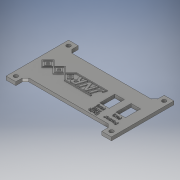
# Autodesk Inventor part: MapleMiniCase_TopCover
Saved by Autodesk Inventor 2018 (Build 220112000, 112)
## iProperties
Created: 2019-01-14
Part Number: MapleMiniCase_TopCover
Material: Generic
Document SubType Name: Modeling
Designer: tbrow
Density: 1 g/cm^3
Appearance: Default
Author: tbrow
## iProperties of the stored document MapleMiniCase_TopCover_3DPrint.ipt
Created: 2019-01-15
Part Number: MapleMiniCase_TopCover_3DPrint
Material: Generic
Document SubType Name: Modeling
Designer: tbrow
Density: 1 g/cm^3
Appearance: Default
Author: tbrow
Autodesk Inventor part; units mm, degrees
ref_plane "YZ Plane" through (0, 0, 0) normal (1, 0, 0) x (0, 1, 0)
ref_plane "XZ Plane" through (0, 0, 0) normal (0, 1, 0) x (-1, 0, 0)
ref_plane "XY Plane" through (0, 0, 0) normal (0, 0, 1) x (1, 0, 0)
sketch "Sketch1" plane through (0, 0, 0) normal (0, 1, 0) x (-1, 0, 0)
  line L0 (0, 0) -> (9.144, 0)
  line L1 (9.144, 0) -> (9.144, -9.144)
  line L2 (9.144, -9.144) -> (89.916, -9.144)
  line L3 (89.916, -9.144) -> (89.916, 0)
  line L4 (89.916, 0) -> (99.06, 0)
  line L5 (99.06, 0) -> (99.06, -58.6994)
  line L6 (99.06, -58.6994) -> (89.916, -58.6994)
  line L7 (89.916, -58.6994) -> (89.916, -49.5554)
  line L8 (89.916, -49.5554) -> (9.144, -49.5554)
  line L9 (9.144, -49.5554) -> (9.144, -58.6994)
  line L10 (9.144, -58.6994) -> (0, -58.6994)
  line L11 (0, -58.6994) -> (0, 0)
  dimension "d0" = 58.6994
  dimension "d1" = 9.144
  dimension "d2" = 9.144
  dimension "d3" = 9.144
  dimension "d4" = 9.144
  dimension "d5" = 9.144
  dimension "d7" = 9.144
  dimension "d16" = 99.06
  constraints: 24 end point, 8 perpendicular, 4 point on line, 2 horizontal
  measures "d0" distance of L4.end L5.end
  measures "d1" distance of L3.end L4.end
  measures "d2" distance of L2.end L3.end
  measures "d3" distance of L6.end L7.end
  measures "d4" distance of L0.start L0.end
  measures "d5" distance of L9.end L10.end
  measures "d7" distance of L5.end L6.end
  measures "d16" distance between parallel lines of L11 L5
extrude "Extrusion1" add sketch "Sketch1" along normal blind 3.175
sketch "Sketch2" plane through (0, 3.175, 0) normal (0, 1, 0) x (1, 0, 0)
  line L0 (-99.06, 0) -> (-89.916, 0) projected
  line L1 (-89.916, 58.6994) -> (-99.06, 58.6994) projected
  line L2 (-89.916, 49.5554) -> (-89.916, 58.6994) projected
  line L3 (-89.916, 0) -> (-89.916, 9.144) projected
  line L4 (-9.144, 0) -> (0, 0) projected
  line L5 (-9.144, 9.144) -> (-9.144, 0) projected
  line L6 (-9.144, 58.6994) -> (-9.144, 49.5554) projected
  circle A0 centre (-94.488, 4.572) radius 1.8542
  circle A1 centre (-94.488, 54.102) radius 1.8542
  circle A2 centre (-4.572, 54.102) radius 1.8542
  circle A3 centre (-4.572, 4.572) radius 1.8542
  line L7 (-99.06, 58.6994) -> (-99.06, 0) projected
  line L8 (0, 58.6994) -> (-9.144, 58.6994) projected
  line L9 (0, 0) -> (0, 58.6994) projected
  dimension "d10" = 3.7084
  dimension "d11" = 3.7084
  dimension "d12" = 3.7084
  dimension "d13" = 3.7084
  dimension "d17" = 4.572
  dimension "d18" = 4.5974
  dimension "d19" = 4.572
  dimension "d20" = 4.572
  dimension "d21" = 4.5974
  dimension "d22" = 4.572
  dimension "d23" = 4.572
  dimension "d24" = 4.572
  constraints: 4 centre point
  measures "d10" diameter of A0
  measures "d11" diameter of A1
  measures "d12" diameter of A2
  measures "d13" diameter of A3
  measures "d17" distance from line of L2 A1.centre
  measures "d18" distance from line of L1 A1.centre
  measures "d19" distance from line of L7 A0.centre
  measures "d20" distance from line of L0 A0.centre
  measures "d21" distance from line of L8 A2.centre
  measures "d22" distance from line of L9 A2.centre
  measures "d23" distance from line of L9 A3.centre
  measures "d24" distance from line of L4 A3.centre
extrude "Extrusion2" cut sketch "Sketch2" against normal blind 25.4
sketch "Sketch3" plane through (0, 3.175, 0) normal (0, 1, 0) x (1, 0, 0)
  line L0 (-33.274, 36.4617) -> (-24.384, 36.4617)
  line L1 (-24.384, 36.4617) -> (-24.384, 22.2377)
  line L2 (-24.384, 22.2377) -> (-33.274, 22.2377)
  line L3 (-33.274, 22.2377) -> (-33.274, 36.4617)
  line L4 (-18.034, 36.4617) -> (-9.144, 36.4617)
  line L5 (-9.144, 36.4617) -> (-9.144, 22.2377)
  line L6 (-9.144, 22.2377) -> (-18.034, 22.2377)
  line L7 (-18.034, 22.2377) -> (-18.034, 36.4617)
  line L8 (0, 0) -> (0, 58.6994) projected
  line L9 (0, 29.3497) -> (-99.06, 29.3497) construction
  line L10 (-99.06, 58.6994) -> (-99.06, 0) projected
  line L11 (-33.274, 29.3497) -> (-24.384, 29.3497) construction
  line L12 (-9.144, 29.3497) -> (-18.034, 29.3497) construction
  dimension "d25" = 14.224
  dimension "d26" = 8.89
  dimension "d27" = 8.89
  dimension "d28" = 6.35
  dimension "d32" = 9.144
  constraints: 22 end point, 6 midpoint, 4 parallel, 2 horizontal, 2 perpendicular, 2 point on line, 1 collinear
  measures "d25" distance of L2.end L0.start
  measures "d26" distance of L0.start L0.end
  measures "d27" distance of L4.start L4.end
  measures "d28" distance between parallel lines of L7 L1
  measures "d32" distance between parallel lines of L8 L5
extrude "Extrusion3" cut sketch "Sketch3" against normal blind 25.4
sketch "Sketch5" plane through (0, 3.175, 0) normal (0, 1, 0) x (1, 0, 0)
  line L0 (-6.9163, 11.6778) -> (-20.2617, 11.6778) construction
  line L1 (-20.2617, 11.6778) -> (-20.2617, 14.6888) construction
  line L2 (-20.2617, 14.6888) -> (-6.9163, 14.6888) construction
  line L3 (-6.9163, 14.6888) -> (-6.9163, 11.6778) construction
  line L4 (-24.384, 22.2377) -> (-33.274, 22.2377) projected
  line L5 (-13.589, 11.6778) -> (-13.589, 11.613) construction
  line L6 (-18.034, 22.2377) -> (-9.144, 22.2377) projected
  line L7 (-13.589, 22.2377) -> (-13.589, 19.0879) construction
  line L8 (-10.6511, 22.2377) -> (-10.6511, 9.144) construction
  line L9 (-89.916, 9.144) -> (-9.144, 9.144) projected
  line L10 (-10.6511, 15.6909) -> (6.071, 15.6909) construction
  line L11 (-24.3341, 10.4275) -> (-33.3239, 10.4275) construction
  line L12 (-33.3239, 10.4275) -> (-33.3239, 17.0935) construction
  line L13 (-33.3239, 17.0935) -> (-24.3341, 17.0935) construction
  line L14 (-24.3341, 17.0935) -> (-24.3341, 10.4275) construction
  line L15 (-33.274, 22.2377) -> (-33.274, 36.4617) projected
  line L16 (-28.829, 10.4275) -> (-28.829, 6.1852) construction
  line L17 (-33.274, 22.2377) -> (-24.384, 22.2377) projected
  line L18 (-28.829, 22.2377) -> (-28.829, 19.0879) construction
  line L19 (-10.5884, 17.4665) -> (-16.5896, 17.4665) construction
  line L20 (-16.5896, 17.4665) -> (-16.5896, 19.3689) construction
  line L21 (-16.5896, 19.3689) -> (-10.5884, 19.3689) construction
  line L22 (-10.5884, 19.3689) -> (-10.5884, 17.4665) construction
  line L23 (-13.589, 17.4665) -> (-13.589, 15.0559) construction
  line L24 (-26.266, 17.4665) -> (-31.392, 17.4665) construction
  line L25 (-31.392, 17.4665) -> (-31.392, 20.1702) construction
  line L26 (-31.392, 20.1702) -> (-26.266, 20.1702) construction
  line L27 (-26.266, 20.1702) -> (-26.266, 17.4665) construction
  line L28 (-28.829, 17.4665) -> (-28.829, 17.4255) construction
  spline S0 degree 2 poles (-9.8961, 12.5585) (-9.8961, 12.7532) (-9.7716, 13.1065) (-9.6561, 13.2242) knots 0 0 0 1 2 2 2
  spline S1 degree 2 poles (-9.6561, 13.2242) (-9.5859, 13.2989) (-9.4138, 13.4212) (-9.312, 13.4642) knots 0 0 0 1 2 2 2
  spline S2 degree 2 poles (-9.312, 13.4642) (-9.2078, 13.5072) (-8.9655, 13.557) (-8.8161, 13.557) knots 0 0 0 1 2 2 2
  line L29 (-8.8161, 13.557) -> (-8.4493, 13.557)
  line L30 (-8.4493, 13.557) -> (-8.4493, 14.4718)
  line L31 (-8.4493, 14.4718) -> (-7.7474, 14.4718)
  line L32 (-7.7474, 14.4718) -> (-7.7474, 11.6778)
  line L33 (-7.7474, 11.6778) -> (-8.832, 11.6778)
  spline S3 degree 2 poles (-8.832, 11.6778) (-9.072, 11.6778) (-9.4229, 11.7661) (-9.5655, 11.8612) knots 0 0 0 1 2 2 2
  spline S4 degree 2 poles (-9.5655, 11.8612) (-9.724, 11.9676) (-9.8961, 12.3163) (-9.8961, 12.5585) knots 0 0 0 1 2 2 2
  spline S5 degree 2 poles (-9.1761, 12.5766) (-9.1761, 12.4566) (-9.0629, 12.2868) (-8.9859, 12.2551) knots 0 0 0 1 2 2 2
  spline S6 degree 2 poles (-8.9859, 12.2551) (-8.8863, 12.2121) (-8.7052, 12.1985) (-8.5489, 12.1985) knots 0 0 0 1 2 2 2
  line L34 (-8.5489, 12.1985) -> (-8.4493, 12.1985)
  line L35 (-8.4493, 12.1985) -> (-8.4493, 13.0363)
  line L36 (-8.4493, 13.0363) -> (-8.4991, 13.0363)
  spline S7 degree 2 poles (-8.4991, 13.0363) (-8.5965, 13.0363) (-8.7731, 13.0317) (-8.8387, 13.0204) knots 0 0 0 1 2 2 2
  spline S8 degree 2 poles (-8.8387, 13.0204) (-8.8954, 13.0114) (-9.0199, 12.957) (-9.0538, 12.9231) knots 0 0 0 1 2 2 2
  spline S9 degree 2 poles (-9.0538, 12.9231) (-9.1263, 12.8551) (-9.1761, 12.7034) (-9.1761, 12.5766) knots 0 0 0 1 2 2 2
  spline S10 degree 2 poles (-12.2554, 13.4189) (-12.2554, 13.9397) (-11.6871, 14.5374) (-11.1686, 14.5374) knots 0 0 0 1 2 2 2
  spline S11 degree 2 poles (-11.1686, 14.5374) (-10.6524, 14.5374) (-10.0795, 13.9397) (-10.0795, 13.4189) knots 0 0 0 1 2 2 2
  spline S12 degree 2 poles (-10.0795, 13.4189) (-10.0795, 12.8936) (-10.6524, 12.2981) (-11.1686, 12.2981) knots 0 0 0 1 2 2 2
  spline S13 degree 2 poles (-11.1686, 12.2981) (-11.6848, 12.2981) (-12.2554, 12.8959) (-12.2554, 13.4189) knots 0 0 0 1 2 2 2
  spline S14 degree 2 poles (-11.5829, 13.4234) (-11.5829, 13.2355) (-11.5218, 12.9842) (-11.4675, 12.9095) knots 0 0 0 1 2 2 2
  spline S15 degree 2 poles (-11.4675, 12.9095) (-11.4086, 12.8302) (-11.2614, 12.7691) (-11.1686, 12.7691) knots 0 0 0 1 2 2 2
  spline S16 degree 2 poles (-11.1686, 12.7691) (-11.078, 12.7691) (-10.9354, 12.8234) (-10.8765, 12.9004) knots 0 0 0 1 2 2 2
  spline S17 degree 2 poles (-10.8765, 12.9004) (-10.8199, 12.9729) (-10.752, 13.2287) (-10.752, 13.4234) knots 0 0 0 1 2 2 2
  spline S18 degree 2 poles (-10.752, 13.4234) (-10.752, 13.6159) (-10.8154, 13.8536) (-10.8675, 13.9261) knots 0 0 0 1 2 2 2
  spline S19 degree 2 poles (-10.8675, 13.9261) (-10.9195, 13.9985) (-11.078, 14.0665) (-11.1731, 14.0665) knots 0 0 0 1 2 2 2
  spline S20 degree 2 poles (-11.1731, 14.0665) (-11.2524, 14.0665) (-11.4154, 13.9985) (-11.4652, 13.9306) knots 0 0 0 1 2 2 2
  spline S21 degree 2 poles (-11.4652, 13.9306) (-11.5218, 13.8514) (-11.5829, 13.6227) (-11.5829, 13.4234) knots 0 0 0 1 2 2 2
  line L37 (-15.7445, 12.3638) -> (-15.1286, 14.4718)
  line L38 (-15.1286, 14.4718) -> (-14.4313, 14.4718)
  line L39 (-14.4313, 14.4718) -> (-14.0599, 13.1087)
  line L40 (-14.0599, 13.1087) -> (-13.6886, 14.4718)
  line L41 (-13.6886, 14.4718) -> (-12.9913, 14.4718)
  line L42 (-12.9913, 14.4718) -> (-12.3799, 12.3638)
  line L43 (-12.3799, 12.3638) -> (-13.0705, 12.3638)
  line L44 (-13.0705, 12.3638) -> (-13.3943, 13.7585)
  line L45 (-13.3943, 13.7585) -> (-13.7928, 12.3638)
  line L46 (-13.7928, 12.3638) -> (-14.3747, 12.3638)
  line L47 (-14.3747, 12.3638) -> (-14.7505, 13.7585)
  line L48 (-14.7505, 13.7585) -> (-15.0698, 12.3638)
  line L49 (-15.0698, 12.3638) -> (-15.7445, 12.3638)
  spline S22 degree 2 poles (-17.103, 14.5284) (-16.5053, 14.5284) (-15.869, 13.9578) (-15.869, 13.4302) knots 0 0 0 1 2 2 2
  spline S23 degree 2 poles (-15.869, 13.4302) (-15.869, 12.914) (-16.4622, 12.2981) (-16.9966, 12.2981) knots 0 0 0 1 2 2 2
  spline S24 degree 2 poles (-16.9966, 12.2981) (-17.4789, 12.2981) (-17.9679, 12.8212) (-17.9679, 13.3057) knots 0 0 0 1 2 2 2
  line L50 (-17.9679, 13.3057) -> (-17.9679, 13.5434)
  line L51 (-17.9679, 13.5434) -> (-16.5256, 13.5434)
  spline S25 degree 2 poles (-16.5256, 13.5434) (-16.5347, 13.6906) (-16.6411, 13.8853) (-16.7272, 13.9442) knots 0 0 0 1 2 2 2
  spline S26 degree 2 poles (-16.7272, 13.9442) (-16.8109, 14.0031) (-17.0373, 14.0529) (-17.1709, 14.0529) knots 0 0 0 1 2 2 2
  spline S27 degree 2 poles (-17.1709, 14.0529) (-17.2841, 14.0529) (-17.506, 14.0031) (-17.5989, 13.9601) knots 0 0 0 1 2 2 2
  spline S28 degree 2 poles (-17.5989, 13.9601) (-17.6804, 13.9261) (-17.8162, 13.8423) (-17.8592, 13.8106) knots 0 0 0 1 2 2 2
  line L52 (-17.8592, 13.8106) -> (-17.9294, 13.8106)
  line L53 (-17.9294, 13.8106) -> (-17.9294, 14.354)
  spline S29 degree 2 poles (-17.9294, 14.354) (-17.8479, 14.3857) (-17.7166, 14.4401) (-17.5989, 14.4672) knots 0 0 0 1 2 2 2
  spline S30 degree 2 poles (-17.5989, 14.4672) (-17.4924, 14.4967) (-17.266, 14.5284) (-17.103, 14.5284) knots 0 0 0 1 2 2 2
  spline S31 degree 2 poles (-17.3204, 13.1472) (-17.3158, 12.9389) (-17.1324, 12.7193) (-16.9445, 12.7193) knots 0 0 0 1 2 2 2
  spline S32 degree 2 poles (-16.9445, 12.7193) (-16.7521, 12.7193) (-16.5347, 12.9502) (-16.5234, 13.1472) knots 0 0 0 1 2 2 2
  line L54 (-16.5234, 13.1472) -> (-17.3204, 13.1472)
  line L55 (-19.7204, 12.9865) -> (-19.6661, 12.9865)
  spline S33 degree 2 poles (-19.6661, 12.9865) (-19.6276, 12.9729) (-19.4849, 12.9593) (-19.3989, 12.9593) knots 0 0 0 1 2 2 2
  spline S34 degree 2 poles (-19.3989, 12.9593) (-19.297, 12.9593) (-19.0683, 13.0204) (-18.9619, 13.0612) knots 0 0 0 1 2 2 2
  line L56 (-18.9619, 13.0612) -> (-18.9619, 14.4718)
  line L57 (-18.9619, 14.4718) -> (-18.3053, 14.4718)
  line L58 (-18.3053, 14.4718) -> (-18.3053, 12.3638)
  line L59 (-18.3053, 12.3638) -> (-18.9619, 12.3638)
  line L60 (-18.9619, 12.3638) -> (-18.9619, 12.6672)
  spline S35 degree 2 poles (-18.9619, 12.6672) (-19.0072, 12.6265) (-19.1657, 12.4997) (-19.2313, 12.4612) knots 0 0 0 1 2 2 2
  spline S36 degree 2 poles (-19.2313, 12.4612) (-19.3038, 12.4181) (-19.494, 12.357) (-19.5778, 12.357) knots 0 0 0 1 2 2 2
  spline S37 degree 2 poles (-19.5778, 12.357) (-19.6095, 12.357) (-19.6887, 12.3615) (-19.7204, 12.3638) knots 0 0 0 1 2 2 2
  line L61 (-19.7204, 12.3638) -> (-19.7204, 12.9865)
  line L62 (-11.1842, 20.3183) -> (-10.6523, 20.3183)
  spline S38 degree 2 poles (-10.6523, 20.3183) (-10.5298, 20.1713) (-10.3286, 19.8616) (-10.2569, 19.6832) knots 0 0 0 1 2 2 2
  spline S39 degree 2 poles (-10.2569, 19.6832) (-10.1887, 19.517) (-10.1117, 19.1111) (-10.1117, 18.8924) knots 0 0 0 1 2 2 2
  spline S40 degree 2 poles (-10.1117, 18.8924) (-10.1117, 18.6527) (-10.1922, 18.2643) (-10.2551, 18.1033) knots 0 0 0 1 2 2 2
  spline S41 degree 2 poles (-10.2551, 18.1033) (-10.3251, 17.9283) (-10.5263, 17.6169) (-10.6523, 17.4665) knots 0 0 0 1 2 2 2
  line L63 (-10.6523, 17.4665) -> (-11.1842, 17.4665)
  line L64 (-11.1842, 17.4665) -> (-11.1842, 17.5084)
  spline S42 degree 2 poles (-11.1842, 17.5084) (-11.067, 17.6134) (-10.8535, 17.8829) (-10.7625, 18.0613) knots 0 0 0 1 2 2 2
  spline S43 degree 2 poles (-10.7625, 18.0613) (-10.675, 18.2345) (-10.5666, 18.6544) (-10.5666, 18.8924) knots 0 0 0 1 2 2 2
  spline S44 degree 2 poles (-10.5666, 18.8924) (-10.5666, 19.1408) (-10.6716, 19.5432) (-10.7625, 19.7234) knots 0 0 0 1 2 2 2
  spline S45 degree 2 poles (-10.7625, 19.7234) (-10.85, 19.8931) (-11.0687, 20.1731) (-11.1842, 20.2763) knots 0 0 0 1 2 2 2
  line L65 (-11.1842, 20.2763) -> (-11.1842, 20.3183)
  spline S46 degree 2 poles (-13.4901, 18.6422) (-13.4901, 19.1671) (-12.9303, 19.7672) (-12.4439, 19.7672) knots 0 0 0 1 2 2 2
  spline S47 degree 2 poles (-12.4439, 19.7672) (-11.9558, 19.7672) (-11.3994, 19.1601) (-11.3994, 18.6422) knots 0 0 0 1 2 2 2
  spline S48 degree 2 poles (-11.3994, 18.6422) (-11.3994, 18.1226) (-11.9558, 17.5172) (-12.4439, 17.5172) knots 0 0 0 1 2 2 2
  spline S49 degree 2 poles (-12.4439, 17.5172) (-12.9303, 17.5172) (-13.4901, 18.1191) (-13.4901, 18.6422) knots 0 0 0 1 2 2 2
  spline S50 degree 2 poles (-12.9303, 18.6422) (-12.9303, 18.448) (-12.8515, 18.1768) (-12.7833, 18.0911) knots 0 0 0 1 2 2 2
  spline S51 degree 2 poles (-12.7833, 18.0911) (-12.7151, 18.0018) (-12.5401, 17.9248) (-12.4456, 17.9248) knots 0 0 0 1 2 2 2
  spline S52 degree 2 poles (-12.4456, 17.9248) (-12.3459, 17.9248) (-12.1832, 17.9966) (-12.108, 18.0876) knots 0 0 0 1 2 2 2
  spline S53 degree 2 poles (-12.108, 18.0876) (-12.0415, 18.1715) (-11.9593, 18.4497) (-11.9593, 18.6422) knots 0 0 0 1 2 2 2
  spline S54 degree 2 poles (-11.9593, 18.6422) (-11.9593, 18.8416) (-12.038, 19.1041) (-12.1062, 19.1933) knots 0 0 0 1 2 2 2
  spline S55 degree 2 poles (-12.1062, 19.1933) (-12.1745, 19.2825) (-12.3512, 19.3595) (-12.4456, 19.3595) knots 0 0 0 1 2 2 2
  spline S56 degree 2 poles (-12.4456, 19.3595) (-12.5419, 19.3595) (-12.7203, 19.2773) (-12.7851, 19.1898) knots 0 0 0 1 2 2 2
  spline S57 degree 2 poles (-12.7851, 19.1898) (-12.855, 19.0953) (-12.9303, 18.8451) (-12.9303, 18.6422) knots 0 0 0 1 2 2 2
  line L66 (-15.6614, 19.7217) -> (-15.14, 19.7217)
  line L67 (-15.14, 19.7217) -> (-14.3072, 18.217)
  line L68 (-14.3072, 18.217) -> (-14.3072, 19.7217)
  line L69 (-14.3072, 19.7217) -> (-13.8121, 19.7217)
  line L70 (-13.8121, 19.7217) -> (-13.8121, 17.5627)
  line L71 (-13.8121, 17.5627) -> (-14.4769, 17.5627)
  line L72 (-14.4769, 17.5627) -> (-15.1663, 18.7996)
  line L73 (-15.1663, 18.7996) -> (-15.1663, 17.5627)
  line L74 (-15.1663, 17.5627) -> (-15.6614, 17.5627)
  line L75 (-15.6614, 17.5627) -> (-15.6614, 19.7217)
  spline S58 degree 2 poles (-17.0628, 18.8924) (-17.0628, 19.1111) (-16.9858, 19.5152) (-16.9176, 19.6832) knots 0 0 0 1 2 2 2
  spline S59 degree 2 poles (-16.9176, 19.6832) (-16.8459, 19.8616) (-16.6447, 20.1713) (-16.5222, 20.3183) knots 0 0 0 1 2 2 2
  line L76 (-16.5222, 20.3183) -> (-15.9903, 20.3183)
  line L77 (-15.9903, 20.3183) -> (-15.9903, 20.2763)
  spline S60 degree 2 poles (-15.9903, 20.2763) (-16.1058, 20.1731) (-16.3262, 19.8949) (-16.412, 19.7234) knots 0 0 0 1 2 2 2
  spline S61 degree 2 poles (-16.412, 19.7234) (-16.503, 19.5432) (-16.6079, 19.1408) (-16.6079, 18.8924) knots 0 0 0 1 2 2 2
  spline S62 degree 2 poles (-16.6079, 18.8924) (-16.6079, 18.6544) (-16.4995, 18.2345) (-16.412, 18.0613) knots 0 0 0 1 2 2 2
  spline S63 degree 2 poles (-16.412, 18.0613) (-16.321, 17.8829) (-16.1075, 17.6134) (-15.9903, 17.5084) knots 0 0 0 1 2 2 2
  line L78 (-15.9903, 17.5084) -> (-15.9903, 17.4665)
  line L79 (-15.9903, 17.4665) -> (-16.5222, 17.4665)
  spline S64 degree 2 poles (-16.5222, 17.4665) (-16.6482, 17.6169) (-16.8494, 17.9283) (-16.9194, 18.1033) knots 0 0 0 1 2 2 2
  spline S65 degree 2 poles (-16.9194, 18.1033) (-16.9823, 18.2643) (-17.0628, 18.6527) (-17.0628, 18.8924) knots 0 0 0 1 2 2 2
  line L80 (-26.4242, 20.3183) -> (-25.8923, 20.3183)
  spline S66 degree 2 poles (-25.8923, 20.3183) (-25.7698, 20.1713) (-25.5686, 19.8616) (-25.4969, 19.6832) knots 0 0 0 1 2 2 2
  spline S67 degree 2 poles (-25.4969, 19.6832) (-25.4287, 19.517) (-25.3517, 19.1111) (-25.3517, 18.8924) knots 0 0 0 1 2 2 2
  spline S68 degree 2 poles (-25.3517, 18.8924) (-25.3517, 18.6527) (-25.4322, 18.2643) (-25.4951, 18.1033) knots 0 0 0 1 2 2 2
  spline S69 degree 2 poles (-25.4951, 18.1033) (-25.5651, 17.9283) (-25.7663, 17.6169) (-25.8923, 17.4665) knots 0 0 0 1 2 2 2
  line L81 (-25.8923, 17.4665) -> (-26.4242, 17.4665)
  line L82 (-26.4242, 17.4665) -> (-26.4242, 17.5084)
  spline S70 degree 2 poles (-26.4242, 17.5084) (-26.307, 17.6134) (-26.0935, 17.8829) (-26.0025, 18.0613) knots 0 0 0 1 2 2 2
  spline S71 degree 2 poles (-26.0025, 18.0613) (-25.915, 18.2345) (-25.8066, 18.6544) (-25.8066, 18.8924) knots 0 0 0 1 2 2 2
  spline S72 degree 2 poles (-25.8066, 18.8924) (-25.8066, 19.1408) (-25.9116, 19.5432) (-26.0025, 19.7234) knots 0 0 0 1 2 2 2
  spline S73 degree 2 poles (-26.0025, 19.7234) (-26.09, 19.8931) (-26.3087, 20.1731) (-26.4242, 20.2763) knots 0 0 0 1 2 2 2
  line L83 (-26.4242, 20.2763) -> (-26.4242, 20.3183)
  spline S74 degree 2 poles (-28.7301, 18.6422) (-28.7301, 19.1671) (-28.1703, 19.7672) (-27.6839, 19.7672) knots 0 0 0 1 2 2 2
  spline S75 degree 2 poles (-27.6839, 19.7672) (-27.1958, 19.7672) (-26.6394, 19.1601) (-26.6394, 18.6422) knots 0 0 0 1 2 2 2
  spline S76 degree 2 poles (-26.6394, 18.6422) (-26.6394, 18.1226) (-27.1958, 17.5172) (-27.6839, 17.5172) knots 0 0 0 1 2 2 2
  spline S77 degree 2 poles (-27.6839, 17.5172) (-28.1703, 17.5172) (-28.7301, 18.1191) (-28.7301, 18.6422) knots 0 0 0 1 2 2 2
  spline S78 degree 2 poles (-28.1703, 18.6422) (-28.1703, 18.448) (-28.0915, 18.1768) (-28.0233, 18.0911) knots 0 0 0 1 2 2 2
  spline S79 degree 2 poles (-28.0233, 18.0911) (-27.9551, 18.0018) (-27.7801, 17.9248) (-27.6856, 17.9248) knots 0 0 0 1 2 2 2
  spline S80 degree 2 poles (-27.6856, 17.9248) (-27.5859, 17.9248) (-27.4232, 17.9966) (-27.348, 18.0876) knots 0 0 0 1 2 2 2
  spline S81 degree 2 poles (-27.348, 18.0876) (-27.2815, 18.1715) (-27.1993, 18.4497) (-27.1993, 18.6422) knots 0 0 0 1 2 2 2
  spline S82 degree 2 poles (-27.1993, 18.6422) (-27.1993, 18.8416) (-27.278, 19.1041) (-27.3462, 19.1933) knots 0 0 0 1 2 2 2
  spline S83 degree 2 poles (-27.3462, 19.1933) (-27.4145, 19.2825) (-27.5912, 19.3595) (-27.6856, 19.3595) knots 0 0 0 1 2 2 2
  spline S84 degree 2 poles (-27.6856, 19.3595) (-27.7819, 19.3595) (-27.9603, 19.2773) (-28.0251, 19.1898) knots 0 0 0 1 2 2 2
  spline S85 degree 2 poles (-28.0251, 19.1898) (-28.095, 19.0953) (-28.1703, 18.8451) (-28.1703, 18.6422) knots 0 0 0 1 2 2 2
  line L84 (-30.9014, 19.7217) -> (-30.38, 19.7217)
  line L85 (-30.38, 19.7217) -> (-29.5472, 18.217)
  line L86 (-29.5472, 18.217) -> (-29.5472, 19.7217)
  line L87 (-29.5472, 19.7217) -> (-29.0521, 19.7217)
  line L88 (-29.0521, 19.7217) -> (-29.0521, 17.5627)
  line L89 (-29.0521, 17.5627) -> (-29.7169, 17.5627)
  line L90 (-29.7169, 17.5627) -> (-30.4063, 18.7996)
  line L91 (-30.4063, 18.7996) -> (-30.4063, 17.5627)
  line L92 (-30.4063, 17.5627) -> (-30.9014, 17.5627)
  line L93 (-30.9014, 17.5627) -> (-30.9014, 19.7217)
  spline S86 degree 2 poles (-32.3028, 18.8924) (-32.3028, 19.1111) (-32.2258, 19.5152) (-32.1576, 19.6832) knots 0 0 0 1 2 2 2
  spline S87 degree 2 poles (-32.1576, 19.6832) (-32.0859, 19.8616) (-31.8847, 20.1713) (-31.7622, 20.3183) knots 0 0 0 1 2 2 2
  line L94 (-31.7622, 20.3183) -> (-31.2303, 20.3183)
  line L95 (-31.2303, 20.3183) -> (-31.2303, 20.2763)
  spline S88 degree 2 poles (-31.2303, 20.2763) (-31.3458, 20.1731) (-31.5662, 19.8949) (-31.652, 19.7234) knots 0 0 0 1 2 2 2
  spline S89 degree 2 poles (-31.652, 19.7234) (-31.743, 19.5432) (-31.8479, 19.1408) (-31.8479, 18.8924) knots 0 0 0 1 2 2 2
  spline S90 degree 2 poles (-31.8479, 18.8924) (-31.8479, 18.6544) (-31.7395, 18.2345) (-31.652, 18.0613) knots 0 0 0 1 2 2 2
  spline S91 degree 2 poles (-31.652, 18.0613) (-31.561, 17.8829) (-31.3475, 17.6134) (-31.2303, 17.5084) knots 0 0 0 1 2 2 2
  line L96 (-31.2303, 17.5084) -> (-31.2303, 17.4665)
  line L97 (-31.2303, 17.4665) -> (-31.7622, 17.4665)
  spline S92 degree 2 poles (-31.7622, 17.4665) (-31.8882, 17.6169) (-32.0894, 17.9283) (-32.1594, 18.1033) knots 0 0 0 1 2 2 2
  spline S93 degree 2 poles (-32.1594, 18.1033) (-32.2223, 18.2643) (-32.3028, 18.6527) (-32.3028, 18.8924) knots 0 0 0 1 2 2 2
  spline S94 degree 2 poles (-27.0584, 11.8268) (-27.0584, 12.2185) (-26.7165, 12.8343) (-26.4561, 12.9996) knots 0 0 0 1 2 2 2
  spline S95 degree 2 poles (-26.4561, 12.9996) (-26.2388, 13.14) (-25.7271, 13.2215) (-25.4395, 13.2215) knots 0 0 0 1 2 2 2
  line L98 (-25.4395, 13.2215) -> (-24.5655, 13.2215)
  line L99 (-24.5655, 13.2215) -> (-24.5655, 10.4275)
  line L100 (-24.5655, 10.4275) -> (-25.4305, 10.4275)
  spline S96 degree 2 poles (-25.4305, 10.4275) (-25.7248, 10.4275) (-26.2388, 10.5022) (-26.4652, 10.6471) knots 0 0 0 1 2 2 2
  spline S97 degree 2 poles (-26.4652, 10.6471) (-26.7392, 10.8237) (-27.0584, 11.4215) (-27.0584, 11.8268) knots 0 0 0 1 2 2 2
  spline S98 degree 2 poles (-26.3384, 11.8222) (-26.3384, 11.546) (-26.1482, 11.152) (-25.9535, 11.0411) knots 0 0 0 1 2 2 2
  spline S99 degree 2 poles (-25.9535, 11.0411) (-25.8108, 10.9641) (-25.4984, 10.9483) (-25.281, 10.9483) knots 0 0 0 1 2 2 2
  line L101 (-25.281, 10.9483) -> (-25.2674, 10.9483)
  line L102 (-25.2674, 10.9483) -> (-25.2674, 12.6985)
  line L103 (-25.2674, 12.6985) -> (-25.281, 12.6985)
  spline S100 degree 2 poles (-25.281, 12.6985) (-25.5165, 12.6985) (-25.8403, 12.6826) (-25.9875, 12.5898) knots 0 0 0 1 2 2 2
  spline S101 degree 2 poles (-25.9875, 12.5898) (-26.1595, 12.4811) (-26.3384, 12.0985) (-26.3384, 11.8222) knots 0 0 0 1 2 2 2
  spline S102 degree 2 poles (-28.5981, 12.9973) (-28.5301, 13.0539) (-28.4237, 13.1445) (-28.3331, 13.1898) knots 0 0 0 1 2 2 2
  spline S103 degree 2 poles (-28.3331, 13.1898) (-28.2448, 13.2328) (-28.0773, 13.2781) (-27.9279, 13.2781) knots 0 0 0 1 2 2 2
  spline S104 degree 2 poles (-27.9279, 13.2781) (-27.6471, 13.2781) (-27.278, 12.9022) (-27.278, 12.617) knots 0 0 0 1 2 2 2
  spline S105 degree 2 poles (-27.278, 12.617) (-27.278, 12.3837) (-27.466, 12.0939) (-27.6426, 12.0102) knots 0 0 0 1 2 2 2
  spline S106 degree 2 poles (-27.6426, 12.0102) (-27.8214, 11.9241) (-28.3173, 11.8562) (-28.6026, 11.8381) knots 0 0 0 1 2 2 2
  line L104 (-28.6026, 11.8381) -> (-28.6026, 11.8268)
  spline S107 degree 2 poles (-28.6026, 11.8268) (-28.6026, 11.6524) (-28.3445, 11.5188) (-28.0863, 11.5188) knots 0 0 0 1 2 2 2
  spline S108 degree 2 poles (-28.0863, 11.5188) (-27.9709, 11.5188) (-27.6584, 11.6026) (-27.5112, 11.6683) knots 0 0 0 1 2 2 2
  line L105 (-27.5112, 11.6683) -> (-27.4546, 11.6683)
  line L106 (-27.4546, 11.6683) -> (-27.4546, 11.1588)
  spline S109 degree 2 poles (-27.4546, 11.1588) (-27.552, 11.1317) (-27.9867, 11.0547) (-28.2086, 11.0547) knots 0 0 0 1 2 2 2
  spline S110 degree 2 poles (-28.2086, 11.0547) (-28.752, 11.0547) (-29.2501, 11.4169) (-29.2501, 11.7883) knots 0 0 0 1 2 2 2
  line L107 (-29.2501, 11.7883) -> (-29.2501, 13.2215)
  line L108 (-29.2501, 13.2215) -> (-28.5981, 13.2215)
  line L109 (-28.5981, 13.2215) -> (-28.5981, 12.9973)
  line L110 (-28.5981, 12.6713) -> (-28.5981, 12.2343)
  spline S111 degree 2 poles (-28.5981, 12.2343) (-28.4305, 12.2502) (-28.2245, 12.2751) (-28.1248, 12.3113) knots 0 0 0 1 2 2 2
  spline S112 degree 2 poles (-28.1248, 12.3113) (-28.0365, 12.3407) (-27.9414, 12.463) (-27.9414, 12.5626) knots 0 0 0 1 2 2 2
  spline S113 degree 2 poles (-27.9414, 12.5626) (-27.9414, 12.7098) (-28.1022, 12.8207) (-28.2584, 12.8207) knots 0 0 0 1 2 2 2
  spline S114 degree 2 poles (-28.2584, 12.8207) (-28.3445, 12.8207) (-28.5256, 12.7415) (-28.5981, 12.6713) knots 0 0 0 1 2 2 2
  spline S115 degree 2 poles (-30.543, 13.2623) (-30.1422, 13.2623) (-29.7754, 12.9317) (-29.7754, 12.5558) knots 0 0 0 1 2 2 2
  line L111 (-29.7754, 12.5558) -> (-29.7754, 11.5709)
  line L112 (-29.7754, 11.5709) -> (-29.5241, 11.5709)
  line L113 (-29.5241, 11.5709) -> (-29.5241, 11.1135)
  line L114 (-29.5241, 11.1135) -> (-29.7754, 11.1135)
  line L115 (-29.7754, 11.1135) -> (-29.7754, 10.5113)
  line L116 (-29.7754, 10.5113) -> (-30.432, 10.5113)
  line L117 (-30.432, 10.5113) -> (-30.432, 11.1135)
  line L118 (-30.432, 11.1135) -> (-31.066, 11.1135)
  line L119 (-31.066, 11.1135) -> (-31.066, 11.5709)
  line L120 (-31.066, 11.5709) -> (-30.432, 11.5709)
  line L121 (-30.432, 11.5709) -> (-30.432, 12.3204)
  spline S116 degree 2 poles (-30.432, 12.3204) (-30.432, 12.4313) (-30.4366, 12.5966) (-30.4637, 12.6622) knots 0 0 0 1 2 2 2
  spline S117 degree 2 poles (-30.4637, 12.6622) (-30.4909, 12.7279) (-30.6245, 12.8049) (-30.7513, 12.8049) knots 0 0 0 1 2 2 2
  spline S118 degree 2 poles (-30.7513, 12.8049) (-30.8056, 12.8049) (-30.9754, 12.7596) (-31.0094, 12.7415) knots 0 0 0 1 2 2 2
  line L122 (-31.0094, 12.7415) -> (-31.066, 12.7415)
  line L123 (-31.066, 12.7415) -> (-31.066, 13.2034)
  spline S119 degree 2 poles (-31.066, 13.2034) (-30.9596, 13.2306) (-30.7196, 13.2623) (-30.543, 13.2623) knots 0 0 0 1 2 2 2
  spline S120 degree 2 poles (-32.4947, 12.9973) (-32.4268, 13.0539) (-32.3204, 13.1445) (-32.2298, 13.1898) knots 0 0 0 1 2 2 2
  spline S121 degree 2 poles (-32.2298, 13.1898) (-32.1415, 13.2328) (-31.9739, 13.2781) (-31.8245, 13.2781) knots 0 0 0 1 2 2 2
  spline S122 degree 2 poles (-31.8245, 13.2781) (-31.5438, 13.2781) (-31.1747, 12.9022) (-31.1747, 12.617) knots 0 0 0 1 2 2 2
  spline S123 degree 2 poles (-31.1747, 12.617) (-31.1747, 12.3837) (-31.3626, 12.0939) (-31.5392, 12.0102) knots 0 0 0 1 2 2 2
  spline S124 degree 2 poles (-31.5392, 12.0102) (-31.7181, 11.9241) (-32.214, 11.8562) (-32.4992, 11.8381) knots 0 0 0 1 2 2 2
  line L124 (-32.4992, 11.8381) -> (-32.4992, 11.8268)
  spline S125 degree 2 poles (-32.4992, 11.8268) (-32.4992, 11.6524) (-32.2411, 11.5188) (-31.983, 11.5188) knots 0 0 0 1 2 2 2
  spline S126 degree 2 poles (-31.983, 11.5188) (-31.8675, 11.5188) (-31.5551, 11.6026) (-31.4079, 11.6683) knots 0 0 0 1 2 2 2
  line L125 (-31.4079, 11.6683) -> (-31.3513, 11.6683)
  line L126 (-31.3513, 11.6683) -> (-31.3513, 11.1588)
  spline S127 degree 2 poles (-31.3513, 11.1588) (-31.4487, 11.1317) (-31.8834, 11.0547) (-32.1053, 11.0547) knots 0 0 0 1 2 2 2
  spline S128 degree 2 poles (-32.1053, 11.0547) (-32.6487, 11.0547) (-33.1468, 11.4169) (-33.1468, 11.7883) knots 0 0 0 1 2 2 2
  line L127 (-33.1468, 11.7883) -> (-33.1468, 13.2215)
  line L128 (-33.1468, 13.2215) -> (-32.4947, 13.2215)
  line L129 (-32.4947, 13.2215) -> (-32.4947, 12.9973)
  line L130 (-32.4947, 12.6713) -> (-32.4947, 12.2343)
  spline S129 degree 2 poles (-32.4947, 12.2343) (-32.3272, 12.2502) (-32.1211, 12.2751) (-32.0215, 12.3113) knots 0 0 0 1 2 2 2
  spline S130 degree 2 poles (-32.0215, 12.3113) (-31.9332, 12.3407) (-31.8381, 12.463) (-31.8381, 12.5626) knots 0 0 0 1 2 2 2
  spline S131 degree 2 poles (-31.8381, 12.5626) (-31.8381, 12.7098) (-31.9989, 12.8207) (-32.1551, 12.8207) knots 0 0 0 1 2 2 2
  spline S132 degree 2 poles (-32.1551, 12.8207) (-32.2411, 12.8207) (-32.4223, 12.7415) (-32.4947, 12.6713) knots 0 0 0 1 2 2 2
  line L131 (-25.2799, 16.0155) -> (-26.2241, 13.2215)
  line L132 (-26.2241, 13.2215) -> (-26.9894, 13.2215)
  line L133 (-26.9894, 13.2215) -> (-27.9335, 16.0155)
  line L134 (-27.9335, 16.0155) -> (-27.2112, 16.0155)
  line L135 (-27.2112, 16.0155) -> (-27.0369, 15.4449)
  line L136 (-27.0369, 15.4449) -> (-26.1584, 15.4449)
  line L137 (-26.1584, 15.4449) -> (-25.9818, 16.0155)
  line L138 (-25.9818, 16.0155) -> (-25.2799, 16.0155)
  line L139 (-26.8829, 14.9377) -> (-26.5976, 14.014)
  line L140 (-26.5976, 14.014) -> (-26.3101, 14.9377)
  line L141 (-26.3101, 14.9377) -> (-26.8829, 14.9377)
  spline S133 degree 2 poles (-29.206, 16.0721) (-28.9456, 16.0721) (-28.5131, 15.9408) (-28.3524, 15.8049) knots 0 0 0 1 2 2 2
  spline S134 degree 2 poles (-28.3524, 15.8049) (-28.1962, 15.6668) (-28.0196, 15.2525) (-28.0196, 14.9717) knots 0 0 0 1 2 2 2
  spline S135 degree 2 poles (-28.0196, 14.9717) (-28.0196, 14.6683) (-28.2097, 14.2449) (-28.375, 14.1091) knots 0 0 0 1 2 2 2
  spline S136 degree 2 poles (-28.375, 14.1091) (-28.5313, 13.9777) (-28.9569, 13.8509) (-29.1879, 13.8509) knots 0 0 0 1 2 2 2
  spline S137 degree 2 poles (-29.1879, 13.8509) (-29.3622, 13.8509) (-29.7109, 13.9324) (-29.8875, 14.0208) knots 0 0 0 1 2 2 2
  line L142 (-29.8875, 14.0208) -> (-29.8875, 14.5823)
  line L143 (-29.8875, 14.5823) -> (-29.8037, 14.5823)
  spline S138 degree 2 poles (-29.8037, 14.5823) (-29.763, 14.5438) (-29.6498, 14.4532) (-29.5818, 14.417) knots 0 0 0 1 2 2 2
  spline S139 degree 2 poles (-29.5818, 14.417) (-29.5094, 14.3762) (-29.3305, 14.3219) (-29.2196, 14.3219) knots 0 0 0 1 2 2 2
  spline S140 degree 2 poles (-29.2196, 14.3219) (-28.9682, 14.3219) (-28.692, 14.6728) (-28.692, 14.9717) knots 0 0 0 1 2 2 2
  spline S141 degree 2 poles (-28.692, 14.9717) (-28.692, 15.2887) (-28.9864, 15.6012) (-29.2309, 15.6012) knots 0 0 0 1 2 2 2
  spline S142 degree 2 poles (-29.2309, 15.6012) (-29.3554, 15.6012) (-29.5411, 15.5445) (-29.609, 15.5038) knots 0 0 0 1 2 2 2
  spline S143 degree 2 poles (-29.609, 15.5038) (-29.6747, 15.4653) (-29.7698, 15.3793) (-29.8037, 15.3453) knots 0 0 0 1 2 2 2
  line L144 (-29.8037, 15.3453) -> (-29.8875, 15.3453)
  line L145 (-29.8875, 15.3453) -> (-29.8875, 15.9091)
  spline S144 degree 2 poles (-29.8875, 15.9091) (-29.8309, 15.934) (-29.6837, 15.9974) (-29.6067, 16.0178) knots 0 0 0 1 2 2 2
  spline S145 degree 2 poles (-29.6067, 16.0178) (-29.5117, 16.0449) (-29.3441, 16.0721) (-29.206, 16.0721) knots 0 0 0 1 2 2 2
  line L146 (-32.1155, 16.7876) -> (-31.4588, 16.7876)
  line L147 (-31.4588, 16.7876) -> (-31.4588, 15.8072)
  spline S146 degree 2 poles (-31.4588, 15.8072) (-31.3887, 15.8638) (-31.2392, 15.9702) (-31.1713, 16.0019) knots 0 0 0 1 2 2 2
  spline S147 degree 2 poles (-31.1713, 16.0019) (-31.0875, 16.0404) (-30.9494, 16.0721) (-30.8317, 16.0721) knots 0 0 0 1 2 2 2
  spline S148 degree 2 poles (-30.8317, 16.0721) (-30.4717, 16.0721) (-30.0505, 15.4766) (-30.0505, 14.9785) knots 0 0 0 1 2 2 2
  spline S149 degree 2 poles (-30.0505, 14.9785) (-30.0505, 14.7023) (-30.1932, 14.297) (-30.3177, 14.1475) knots 0 0 0 1 2 2 2
  spline S150 degree 2 poles (-30.3177, 14.1475) (-30.4332, 14.0094) (-30.7592, 13.8509) (-30.9403, 13.8509) knots 0 0 0 1 2 2 2
  spline S151 degree 2 poles (-30.9403, 13.8509) (-31.0966, 13.8509) (-31.3275, 13.9302) (-31.4543, 14.0026) knots 0 0 0 1 2 2 2
  line L148 (-31.4543, 14.0026) -> (-31.4792, 13.9075)
  line L149 (-31.4792, 13.9075) -> (-32.1155, 13.9075)
  line L150 (-32.1155, 13.9075) -> (-32.1155, 16.7876)
  line L151 (-31.4588, 15.4336) -> (-31.4588, 14.4011)
  spline S152 degree 2 poles (-31.4588, 14.4011) (-31.4113, 14.3762) (-31.2528, 14.3445) (-31.1962, 14.3445) knots 0 0 0 1 2 2 2
  spline S153 degree 2 poles (-31.1962, 14.3445) (-30.9607, 14.3445) (-30.723, 14.6751) (-30.723, 14.9717) knots 0 0 0 1 2 2 2
  spline S154 degree 2 poles (-30.723, 14.9717) (-30.723, 15.2819) (-30.9132, 15.5604) (-31.1237, 15.5604) knots 0 0 0 1 2 2 2
  spline S155 degree 2 poles (-31.1237, 15.5604) (-31.2098, 15.5604) (-31.3864, 15.4925) (-31.4588, 15.4336) knots 0 0 0 1 2 2 2
  point P0 (0, 0)
  dimension "d34" = 270
  dimension "d35" = 270
  dimension "d36" = 270
  constraints: 16 end point, 7 midpoint, 7 vertical, 5 collinear, 2 point on line, 1 horizontal, 8 other
emboss "Emboss1" sketch "Sketch5" operation add depth 0.508 direction (0, -1, 0)
sketch "Sketch6" plane through (0, 3.175, 0) normal (0, 1, 0) x (1, 0, 0)
  line L0 (-40.3703, 23.4244) -> (-65.0308, 23.4244)
  line L1 (-67.6978, 24.2626) -> (-40.3703, 24.2626)
  line L2 (-40.3703, 24.2626) -> (-40.3703, 23.4244)
  line L3 (-56.7722, 24.8976) -> (-54.7334, 24.8976) construction
  line L4 (-37.8303, 42.2014) -> (-37.8303, 16.4839) construction
  line L5 (-37.2178, 34.4226) -> (-67.6978, 34.4226)
  line L6 (-67.6978, 34.4226) -> (-67.6978, 35.2481) construction
  line L7 (-67.6978, 35.2481) -> (-37.2178, 35.2481)
  line L8 (-37.2178, 35.2481) -> (-37.2178, 34.4226)
  line L9 (-51.6068, 33.7876) -> (-53.7536, 33.7876) construction
  line L10 (-64.8178, 29.3426) -> (-67.9608, 26.1995)
  line L11 (-67.9608, 26.1995) -> (-71.1039, 29.3426)
  line L12 (-71.1039, 29.3426) -> (-67.9608, 32.4857)
  line L13 (-67.9608, 32.4857) -> (-64.8178, 29.3426)
  line L14 (-67.9608, 26.1995) -> (-67.9608, 32.4857) construction
  line L15 (-69.4875, 29.3426) -> (-67.9608, 27.816)
  line L16 (-67.9608, 27.816) -> (-66.4342, 29.3426)
  line L17 (-66.4342, 29.3426) -> (-67.9608, 30.8693)
  line L18 (-67.9608, 30.8693) -> (-69.4875, 29.3426)
  line L19 (-65.0308, 23.4244) -> (-67.9608, 23.4244)
  line L20 (-67.6978, 35.2481) -> (-67.9609, 35.2481)
  line L21 (-73.2268, 28.6904) -> (-73.2268, 24.4371) construction
  line L22 (-81.6359, 29.3426) -> (-78.4928, 26.1995)
  line L23 (-78.4928, 27.816) -> (-80.0195, 29.3426)
  line L24 (-76.9662, 29.3426) -> (-78.4928, 27.816)
  line L25 (-78.4928, 26.1995) -> (-75.3497, 29.3426)
  line L26 (-75.3497, 29.3426) -> (-78.4928, 32.4857)
  line L27 (-78.4928, 30.8693) -> (-76.9662, 29.3426)
  line L28 (-80.0195, 29.3426) -> (-78.4928, 30.8693)
  line L29 (-78.4928, 32.4857) -> (-81.6359, 29.3426)
  line L30 (-83.7588, 28.6904) -> (-83.7588, 23.2318) construction
  line L31 (-85.8817, 29.3426) -> (-89.0248, 26.1995)
  line L32 (-89.0248, 26.1995) -> (-92.1679, 29.3426)
  line L33 (-90.5514, 29.3426) -> (-89.0248, 27.816)
  line L34 (-89.0248, 27.816) -> (-87.4982, 29.3426)
  line L35 (-92.1679, 29.3426) -> (-89.0248, 32.4857)
  line L36 (-89.0248, 30.8693) -> (-90.5514, 29.3426)
  line L37 (-87.4982, 29.3426) -> (-89.0248, 30.8693)
  line L38 (-89.0248, 32.4857) -> (-85.8817, 29.3426)
  line L39 (-88.9961, 24.5544) -> (-93.7843, 29.3426)
  line L40 (-89.0355, 23.4137) -> (-94.9581, 29.3363)
  line L41 (-88.9961, 34.1309) -> (-93.7843, 29.3426)
  line L42 (-89.0355, 35.2589) -> (-94.9581, 29.3363)
  line L43 (-78.4928, 35.2481) -> (-83.7588, 29.9821)
  line L44 (-84.2078, 29.3426) -> (-88.9961, 24.5544)
  line L45 (-78.4928, 34.1596) -> (-83.3098, 29.3426)
  line L46 (-83.7588, 28.6904) -> (-89.0355, 23.4137)
  line L47 (-78.4928, 24.5257) -> (-83.3098, 29.3426)
  line L48 (-83.7588, 29.9821) -> (-89.0355, 35.2589)
  line L49 (-78.4928, 23.4244) -> (-83.7588, 28.6904)
  line L50 (-84.2078, 29.3426) -> (-88.9961, 34.1309)
  line L51 (-67.9608, 23.4244) -> (-73.2268, 28.6904)
  line L52 (-73.6759, 29.3426) -> (-78.4928, 34.1596)
  line L53 (-67.6978, 24.2626) -> (-72.7778, 29.3426)
  line L54 (-73.2268, 29.9821) -> (-78.4928, 35.2481)
  line L55 (-67.6978, 34.4226) -> (-72.7778, 29.3426)
  line L56 (-73.2268, 28.6904) -> (-78.4928, 23.4244)
  line L57 (-67.9609, 35.2481) -> (-73.2268, 29.9821)
  line L58 (-73.6759, 29.3426) -> (-78.4928, 24.5257)
  line L59 (-89.916, 58.6994) -> (-99.06, 58.6994) projected
  line L60 (-33.274, 22.2377) -> (-33.274, 36.4617) projected
  line L61 (-44.2866, 24.2626) -> (-44.2866, 34.4226) construction
  line L62 (-44.2866, 29.3426) -> (-40.1094, 29.3426) construction
  line L63 (-33.274, 29.3497) -> (-111.4558, 29.3497) construction
  line L64 (-39.2583, 25.0026) -> (-65.7075, 25.0026) construction
  line L65 (-65.7075, 25.0026) -> (-65.7075, 34.711) construction
  line L66 (-65.7075, 34.711) -> (-39.2583, 34.711) construction
  line L67 (-39.2583, 34.711) -> (-39.2583, 25.0026) construction
  line L68 (-89.916, 9.144) -> (-9.144, 9.144) projected
  line L69 (-53.5411, 25.0026) -> (-53.5411, 24.2626) construction
  spline S0 degree 2 poles (-45.1794, 30.363) (-44.5774, 32.1525) (-42.2766, 34.0493) (-40.7097, 34.0493) knots 0 0 0 1 2 2 2
  spline S1 degree 2 poles (-40.7097, 34.0493) (-40.0087, 34.0493) (-39.4892, 33.8019) knots 0 0 0 1 1 1
  line L70 (-39.4892, 33.8019) -> (-40.1324, 31.9299)
  spline S2 degree 2 poles (-40.1324, 31.9299) (-40.5118, 32.3175) (-41.155, 32.3175) knots 0 0 0 1 1 1
  spline S3 degree 2 poles (-41.155, 32.3175) (-42.524, 32.3175) (-43.2167, 30.2805) knots 0 0 0 1 1 1
  line L71 (-43.2167, 30.2805) -> (-45.0062, 25.0026)
  line L72 (-45.0062, 25.0026) -> (-47.002, 25.0026)
  line L73 (-47.002, 25.0026) -> (-45.1794, 30.363)
  line L74 (-53.9292, 33.8926) -> (-51.9088, 33.8926)
  line L75 (-51.9088, 33.8926) -> (-50.144, 28.3013)
  spline S4 degree 2 poles (-50.144, 28.3013) (-49.9873, 27.8147) (-49.9461, 27.5673) knots 0 0 0 1 1 1
  line L76 (-49.9461, 27.5673) -> (-49.9213, 27.5673)
  spline S5 degree 2 poles (-49.9213, 27.5673) (-49.8141, 28.0374) (-49.4842, 29.0023) knots 0 0 0 1 1 1
  line L77 (-49.4842, 29.0023) -> (-47.8266, 33.8926)
  line L78 (-47.8266, 33.8926) -> (-45.9299, 33.8926)
  line L79 (-45.9299, 33.8926) -> (-48.9564, 25.0026)
  line L80 (-48.9564, 25.0026) -> (-51.1088, 25.0026)
  line L81 (-51.1088, 25.0026) -> (-52.7994, 30.4125)
  spline S6 degree 2 poles (-52.7994, 30.4125) (-52.9149, 30.7836) (-52.9974, 31.1382) knots 0 0 0 1 1 1
  line L82 (-52.9974, 31.1382) -> (-53.0221, 31.1382)
  spline S7 degree 2 poles (-53.0221, 31.1382) (-53.0798, 30.833) (-53.3932, 29.9177) knots 0 0 0 1 1 1
  line L83 (-53.3932, 29.9177) -> (-55.059, 25.0026)
  line L84 (-55.059, 25.0026) -> (-56.9558, 25.0026)
  line L85 (-56.9558, 25.0026) -> (-53.9292, 33.8926)
  line L86 (-63.4295, 33.8926) -> (-61.1287, 33.8926)
  line L87 (-61.1287, 33.8926) -> (-60.5266, 31.6082)
  spline S8 degree 2 poles (-60.5266, 31.6082) (-60.4607, 31.3443) (-60.3122, 30.932) (-60.1143, 30.6434) (-59.8504, 30.4867) (-59.669, 30.4867) knots 0 0 0 1 2 3 4 4 4
  line L88 (-59.669, 30.4867) -> (-59.1329, 30.4867)
  line L89 (-59.1329, 30.4867) -> (-57.9701, 33.8926)
  line L90 (-57.9701, 33.8926) -> (-55.9662, 33.8926)
  line L91 (-55.9662, 33.8926) -> (-58.9927, 25.0026)
  line L92 (-58.9927, 25.0026) -> (-62.1677, 25.0026)
  spline S9 degree 2 poles (-62.1677, 25.0026) (-65.4005, 25.0026) (-64.584, 27.4189) knots 0 0 0 1 1 1
  spline S10 degree 2 poles (-64.584, 27.4189) (-64.4191, 27.8807) (-63.8666, 28.6724) (-63.1326, 29.3074) (-62.242, 29.761) (-61.7472, 29.8929) knots 0 0 0 1 2 3 4 4 4
  line L93 (-61.7472, 29.8929) -> (-61.7389, 29.9177)
  spline S11 degree 2 poles (-61.7389, 29.9177) (-61.9121, 29.9836) (-62.1925, 30.2558) (-62.4069, 30.6269) (-62.5801, 31.0557) (-62.6461, 31.2619) knots 0 0 0 1 2 3 4 4 4
  line L94 (-62.6461, 31.2619) -> (-63.4295, 33.8926)
  line L95 (-60.4854, 26.5035) -> (-59.6442, 28.9775)
  line L96 (-59.6442, 28.9775) -> (-60.5101, 28.9775)
  spline S12 degree 2 poles (-60.5101, 28.9775) (-61.1534, 28.9775) (-61.6729, 28.6064) knots 0 0 0 1 1 1
  spline S13 degree 2 poles (-61.6729, 28.6064) (-62.2007, 28.2271) (-62.3904, 27.6663) knots 0 0 0 1 1 1
  spline S14 degree 2 poles (-62.3904, 27.6663) (-62.7862, 26.5035) (-61.3925, 26.5035) knots 0 0 0 1 1 1
  line L97 (-61.3925, 26.5035) -> (-60.4854, 26.5035)
  point P0 (0, 0)
  dimension "d39" = 0.8382
  dimension "d40" = 0.635
  dimension "d41" = 2.54
  dimension "d42" = 30.48
  dimension "d43" = 0.635
  dimension "d44" = 0.8255
  dimension "d45" = 45
  dimension "d46" = 10.16
  dimension "d47" = 5.08
  dimension "d48" = 4.445
  dimension "d49" = 4.445
  dimension "d50" = 26.9875
  dimension "d51" = 1.143
  dimension "d52" = 0.8345
  dimension "d53" = 1.143
  dimension "d54" = 0.8255
  dimension "d55" = 1.143
  dimension "d56" = 0
  dimension "d59" = 270
  constraints: 126 end point, 35 parallel, 16 symmetric about line, 5 perpendicular, 4 point on line, 2 horizontal, 2 midpoint, 5 other
  measures "d39" distance of L1.end L0.start
  measures "d40" distance between parallel lines of L1 L3
  measures "d41" distance between parallel lines of L4 L2
  measures "d42" distance of L20.start L7.end
  measures "d43" distance between parallel lines of L5 L9
  measures "d44" distance of L55.start L20.start
  measures "d45" angle of L5 L13
  measures "d46" distance between parallel lines of L5 L1
  measures "d47" distance from line of L1 L13.end
  measures "d48" distance of L13.end L14.start
  measures "d49" distance of L12.end L13.end
  measures "d50" distance from line of L4 L13.end
  measures "d51" distance between parallel lines of L11 L15
  measures "d52" distance between parallel lines of L40 L39
  measures "d53" distance between parallel lines of L39 L32
  measures "d54" distance between parallel lines of L42 L41
  measures "d55" distance between parallel lines of L35 L41
  measures "d56" horizontal distance of L19.end L14.start
emboss "Emboss2" sketch "Sketch6" operation add depth 0.762 direction (0, -1, 0)
sketch "Sketch7" plane through (0, 3.175, 0) normal (0, 1, 0) x (1, 0, 0)
  line L0 (-40.1324, 31.9299) -> (-39.4892, 33.8019) projected
  line L1 (-40.1324, 31.9299) -> (-44.2029, 20.0837)
  line L2 (-39.4892, 33.8019) -> (-37.418, 39.8295)
  line L3 (-37.418, 39.8295) -> (-35.9996, 37.5718)
  line L4 (-35.9996, 37.5718) -> (-36.7079, 19.7852)
  line L5 (-36.7079, 19.7852) -> (-44.2029, 20.0837)
  point P0 (0, 0)
  constraints: 10 end point, 2 collinear, 1 perpendicular
extrude "Extrusion4" cut sketch "Sketch7" along normal blind 25.4
chamfer "Chamfer1" distance 3.175 angle 45 4 edges at (-89.916, 1.5875, -49.5554) (-9.144, 1.5875, -49.5554) (-9.144, 1.5875, -9.144) (-89.916, 1.5875, -9.144)
equation "\"d2\" = d1"
equation "\"d3\" = d1"
equation "\"d4\" = d1"
equation "\"d5\" = d1"
equation "\"d7\" = d1"
equation "\"d19\" = d17"
equation "\"d20\" = d17"
equation "\"d22\" = d17"
equation "\"d23\" = d17"
equation "\"d24\" = d17"
body "Solid1"
